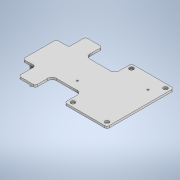
# Autodesk Inventor part: Arduino-ondersteuning
Saved by Autodesk Inventor 2022 (Build 260153000, 153)
## iProperties
Created: 2022-10-19
Part Number: Arduino-ondersteuning
Material: Generic
Document SubType Name: Modeling
Designer: gebruiker
Density: 1 g/cm^3
Appearance: Default
Author: gebruiker
Autodesk Inventor part; units mm, degrees
ref_plane "YZ Plane" through (0, 0, 0) normal (1, 0, 0) x (0, 1, 0)
ref_plane "XZ Plane" through (0, 0, 0) normal (0, 1, 0) x (-1, 0, 0)
ref_plane "XY Plane" through (0, 0, 0) normal (0, 0, 1) x (1, 0, 0)
sketch "Sketch1" plane through (0, 0, 0) normal (0, 1, 0) x (-1, 0, 0)
  line L0 (0, 0) -> (50.75, 0)
  line L1 (50.75, 0) -> (50.75, -80)
  line L2 (50.75, -80) -> (0, -80)
  line L3 (0, -80) -> (0, 0)
  dimension "d0" = 50.75
  dimension "d1" = 80
  constraints: 8 end point, 2 parallel, 1 horizontal, 1 perpendicular
  measures "d0" distance of L1.end L2.end
  measures "d1" distance of L0.end L1.end
extrude "Extrusion1" add sketch "Sketch1" along normal blind 2.5
sketch "Sketch2" plane through (0, 2.5, 0) normal (0, 1, 0) x (1, 0, 0)
  circle A0 centre (-5, 5) radius 2.5
  circle A1 centre (-45.75, 5) radius 2.5
  circle A2 centre (-45.75, 75) radius 2.5
  circle A3 centre (-5, 75) radius 2.5
  line L0 (0, 0) -> (0, 80) projected
  line L1 (-50.75, 0) -> (0, 0) projected
  line L2 (-50.75, 80) -> (-50.75, 0) projected
  line L3 (0, 80) -> (-50.75, 80) projected
  dimension "d4" = 5
  dimension "d5" = 5
  dimension "d6" = 5
  dimension "d7" = 5
  dimension "d8" = 5
  dimension "d9" = 5
  dimension "d10" = 5
  dimension "d11" = 5
  dimension "d12" = 5
  dimension "d13" = 5
  dimension "d14" = 5
  dimension "d15" = 5
  constraints: 4 centre point
  measures "d4" diameter of A0
  measures "d5" diameter of A1
  measures "d6" diameter of A2
  measures "d7" diameter of A3
  measures "d8" distance from line of A0.centre L0
  measures "d9" distance from line of A0.centre L1
  measures "d10" distance from line of A1.centre L1
  measures "d11" distance from line of A1.centre L2
  measures "d12" distance from line of A2.centre L2
  measures "d13" distance from line of L3 A2.centre
  measures "d14" distance from line of L0 A3.centre
  measures "d15" distance from line of A3.centre L3
extrude "Extrusion2" cut sketch "Sketch2" against normal blind 2.5 contours A0 | A1 | A2 | A3
fillet "Fillet1" radius 2.5 4 edges at (-50.75, 1.25, -80) (-50.75, 1.25, 0) (0, 1.25, 0) (0, 1.25, -80)
sketch "Sketch6" plane through (0, 2.5, 0) normal (0, 1, 0) x (1, 0, 0)
  line L0 (-50.75, 60) -> (-120.75, 60)
  line L1 (-120.75, 60) -> (-120.75, 20)
  line L2 (-120.75, 20) -> (-50.75, 20)
  line L3 (-50.75, 20) -> (-50.75, 60)
  line L4 (-2.5, 80) -> (-48.25, 80) projected
  line L5 (-48.25, 0) -> (0, 0) projected
  line L6 (-50.75, 77.5) -> (-50.75, 2.5) projected
  point P0 (0, 80)
  dimension "d64" = 70
  dimension "d65" = 40
  dimension "d68" = 20
  dimension "d69" = 20
  dimension "d72" = 0
  constraints: 8 end point, 2 parallel, 1 horizontal, 1 perpendicular
  measures "d64" distance of L2.end L1.end
  measures "d65" distance of L1.end L0.end
  measures "d68" distance between parallel lines of L0 L4
  measures "d69" distance between parallel lines of L5 L2
  measures "d72" distance between parallel lines of L3 L6
extrude "Extrusion6" add sketch "Sketch6" against normal blind 2.5
sketch "Sketch8" plane through (0, 0, 0) normal (0, -1, 0) x (1, 0, 0)
  line L0 (-110.75, -60) -> (-110.75, -20)
  line L1 (-110.75, -20) -> (-113.25, -20)
  line L2 (-110.75, -60) -> (-110.75, -20)
  line L3 (-120.75, -20) -> (-120.75, -60) projected
  line L4 (-113.25, -20) -> (-113.25, -60)
  line L5 (-120.75, -60) -> (-50.75, -60) projected
  line L6 (-110.75, -60) -> (-113.25, -60)
  point P0 (0, 0)
  dimension "d80" = 2.5
  dimension "d93" = 7.5
  constraints: 10 end point, 1 perpendicular, 1 point on line, 1 vertical
  measures "d80" distance of L1.end L0.end
  measures "d93" distance between parallel lines of L3 L4
extrude "Extrusion8" add sketch "Sketch8" along normal blind 21.5
fillet "Fillet3" radius 1.25 4 edges at (-110.75, -10.75, -20) (-113.25, -10.75, -20) (-113.25, -10.75, -60) (-110.75, -10.75, -60)
fillet "Fillet4" radius 5 2 edges at (-50.75, 1.25, -20) (-50.75, 1.25, -60)
sketch "Sketch11" plane through (-120.75, 0, -20) normal (0, 0, 1) x (1, 0, 0)
  line L0 (65, 2.5) -> (65, 0) projected
  line L1 (0, 2.5) -> (65, 2.5) projected
  line L2 (65, 0) -> (8.75, 0) projected
  line L3 (15, 2.5) -> (35, 2.5)
  line L4 (35, 2.5) -> (35, 0)
  line L5 (35, 0) -> (15, 0)
  line L6 (15, 0) -> (15, 2.5)
  line L7 (0, 2.5) -> (0, 0) projected
  point P0 (120.75, 0)
  dimension "d104" = 20
  dimension "d105" = 15
  dimension "d106" = 30
  constraints: 8 end point, 2 parallel, 2 point on line, 1 horizontal, 1 perpendicular
  measures "d104" distance of L4.end L5.end
  measures "d105" distance between parallel lines of L6 L7
  measures "d106" distance from line of L0 L4.end
extrude "Extrusion11" add sketch "Sketch11" along normal blind 20 contours L4 L2 L6 L1
sketch "Sketch12" plane through (-120.75, 0, -60) normal (0, 0, -1) x (-1, 0, 0)
  line L0 (-15, 0) -> (-35, 0) projected
  line L1 (-35, 2.5) -> (-15, 2.5) projected
  line L2 (-15, 0) -> (-35, 0)
  line L3 (-35, 0) -> (-35, 2.5)
  line L4 (-35, 2.5) -> (-15, 2.5)
  line L5 (-15, 2.5) -> (-15, 0)
  line L6 (0, 2.5) -> (0, 0) projected
  line L7 (-65, 0) -> (-65, 2.5) projected
  point P0 (-120.75, 0)
  dimension "d107" = 15
  dimension "d108" = 30
  constraints: 8 end point, 2 parallel, 1 horizontal, 1 perpendicular
  measures "d107" distance between parallel lines of L6 L5
  measures "d108" distance between parallel lines of L3 L7
extrude "Extrusion12" add sketch "Sketch12" along normal blind 20
fillet "Fillet5" radius 2.5 8 edges at (-105.75, 1.25, -80) (-85.75, 1.25, -80) (-105.75, 1.25, -60) (-120.75, 1.25, -60) (-120.75, 1.25, -20) (-105.75, 1.25, -20) (-85.75, 1.25, 0) (-105.75, 1.25, 0)
fillet "Fillet6" radius 5 2 edges at (-85.75, 1.25, -60) (-85.75, 1.25, -20)
sketch "Sketch13" plane through (0, 2.5, 0) normal (0, 1, 0) x (1, 0, 0)
  circle A0 centre (-65.5, 30) radius 1
  line L0 (-50.75, 15) -> (-50.75, 2.5) projected
  line L1 (-80.75, 20) -> (-55.75, 20) projected
  line L2 (-48.25, 0) -> (-2.5, 0) projected
  circle A1 centre (-14, 63) radius 1
  line L3 (-2.5, 80) -> (-48.25, 80) projected
  line L4 (0, 2.5) -> (0, 77.5) projected
  point P0 (0, 0)
  dimension "d111" = 2
  dimension "d112" = 14.75
  dimension "d113" = 10
  dimension "d114" = 30
  dimension "d124" = 2
  dimension "d125" = 17
  dimension "d126" = 14
  constraints: 2 centre point
  measures "d111" diameter of A0
  measures "d112" distance from line of L0 A0.centre
  measures "d113" distance from line of L1 A0.centre
  measures "d114" distance from line of A0.centre L2
  measures "d124" diameter of A1
  measures "d125" distance from line of A1.centre L3
  measures "d126" distance from line of A1.centre L4
extrude "Extrusion13" cut sketch "Sketch13" against normal blind 20
body "Solid1"
